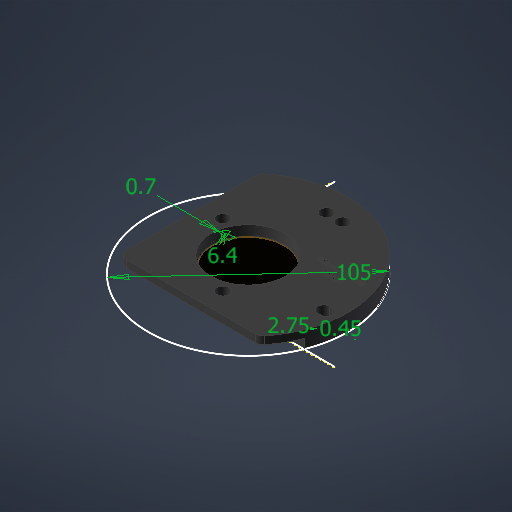
# Autodesk Inventor part: 40x4.35mm Coin Fixture Makera Air V2
Saved by Autodesk Inventor 2026.1 (Build 301233020, 233B)
## iProperties
Created: 2026-01-16
Part Number: 40x4.35mm Coin Fixture Makera Air V2
Material: Generic
Document SubType Name: Modeling
Designer: incep
Density: 1 g/cm^3
Appearance: Default
Author: incep
## iProperties of the stored document 40x4.35mm Coin Fixture Makera Air_3DPrint.ipt
Created: 2026-01-16
Part Number: 40x4.35mm Coin Fixture Makera Air_3DPrint
Material: Generic
Document SubType Name: Modeling
Designer: incep
Density: 1 g/cm^3
Appearance: Default
Author: incep
Autodesk Inventor part; units mm, degrees
ref_plane "YZ Plane" through (0, 0, 0) normal (1, 0, 0) x (0, 1, 0)
ref_plane "XZ Plane" through (0, 0, 0) normal (0, 1, 0) x (-1, 0, 0)
ref_plane "XY Plane" through (0, 0, 0) normal (0, 0, 1) x (1, 0, 0)
sketch "Sketch1" plane through (0, 0, 0) normal (0, 1, 0) x (-1, 0, 0)
  line L0 (0, -85) -> (15, -85) construction
  line L1 (15, -85) -> (15, 15) construction
  line L2 (15, 15) -> (-85, 15) construction
  line L3 (-85, 15) -> (-85, 0) construction
  arc A0 (0, -34.3692) -> (0, -25.6308) centre (3, -30) ccw construction
  arc A1 (-25.6308, 0) -> (-34.3692, 0) centre (-30, 3) ccw construction
  line L4 (0, 0) -> (0, -25.6308) construction
  line L5 (0, -34.3692) -> (0, -85) construction
  line L6 (-85, 0) -> (-34.3692, 0) construction
  line L7 (-25.6308, 0) -> (0, 0) construction
  circle A2 centre (-20.1, -20.1) radius 20.1 construction
  circle A3 centre (-30, -60) radius 1.375 construction
  circle A4 centre (-65, -15) radius 1.375 construction
  circle A5 centre (-66.5, -15) radius 1.375 construction
  circle A6 centre (-21.5, -60) radius 1.375 construction
  dimension "d0" = 85
  dimension "d1" = 15
  dimension "d2" = 100
  dimension "d3" = 100
  dimension "d4" = 15
  dimension "d5" = 85
  dimension "d6" = 10.6
  dimension "d7" = 3
  dimension "d8" = 30
  dimension "d9" = 10.6
  dimension "d10" = 3
  dimension "d11" = 30
  dimension "d12" = 40.2
  dimension "d13" = 2.75
  dimension "d14" = 2.75
  dimension "d15" = 30
  dimension "d16" = 60
  dimension "d17" = 65
  dimension "d18" = 15
  dimension "d49" = 2.75
  dimension "d50" = 2.75
  dimension "d51" = 18
  dimension "d52" = 36.5
  dimension "d53" = 8.5
  dimension "d54" = 63
  constraints: 16 end point, 7 centre point, 5 perpendicular, 4 point on circle, 2 collinear, 2 tangent, 2 vertical
  measures "d0" distance of L4.start L0.start
  measures "d1" distance of L0.start L0.end
  measures "d2" distance of L0.end L1.end
  measures "d3" distance of L1.end L2.end
  measures "d4" distance of L2.end L3.end
  measures "d5" distance of L3.end L4.start
  measures "d6" diameter of A0
  measures "d7" horizontal distance of L4.start A0.centre
  measures "d8" vertical distance of L4.start A0.centre
  measures "d9" diameter of A1
  measures "d10" vertical distance of A1.centre L4.start
  measures "d11" horizontal distance of A1.centre L4.start
  measures "d12" diameter of A2
  measures "d13" diameter of A3
  measures "d14" diameter of A4
  measures "d15" horizontal distance of L4.start A3.centre
  measures "d16" vertical distance of L4.start A3.centre
  measures "d17" horizontal distance of L4.start A4.centre
  measures "d18" vertical distance of L4.start A4.centre
  measures "d49" diameter of A5
  measures "d50" diameter of A6
  measures "d51" vertical distance of A5.centre A1.centre
  measures "d52" horizontal distance of A5.centre A1.centre
  measures "d53" horizontal distance of A1.centre A6.centre
  measures "d54" vertical distance of A1.centre A6.centre
sketch "Sketch2" plane through (0, 0, 0) normal (0, 1, 0) x (-1, 0, 0)
  line L0 (0, 0) -> (0, -25.6308) construction
  line L1 (-25.6308, 0) -> (0, 0) construction
  circle A0 centre (-20.1, -20.1) radius 20.1 projected
  arc A1 (-25.6308, 0) -> (-34.3692, 0) centre (-30, 3) ccw construction
  line L2 (-85, 0) -> (-34.3692, 0) construction
  arc A2 (0, -34.3692) -> (0, -25.6308) centre (3, -30) ccw construction
  line L3 (0, -34.3692) -> (0, -85) construction
  line L4 (-85, -0.7) -> (-32.7331, -0.7)
  arc A3 (-27.2669, -0.7) -> (-32.7331, -0.7) centre (-30, 3) ccw
  line L5 (-27.2669, -0.7) -> (-0.7, -0.7)
  line L6 (-0.7, -0.7) -> (-0.7, -27.2669)
  arc A4 (-0.7, -32.7331) -> (-0.7, -27.2669) centre (3, -30) ccw
  line L7 (-0.7, -32.7331) -> (-0.7, -85)
  circle A5 centre (-20.1, -20.1) radius 52.5
  circle A6 centre (-30, -60) radius 1.375 construction
  circle A7 centre (-65, -15) radius 1.375 construction
  circle A8 centre (3, -30) radius 3.2
  circle A9 centre (-30, 3) radius 3.2
  circle A10 centre (-65, -15) radius 3.2 construction
  circle A11 centre (-30, -60) radius 3.2
  circle A12 centre (-21.5, -60) radius 1.375 construction
  circle A13 centre (-66.5, -15) radius 1.375 construction
  circle A14 centre (-21.5, -60) radius 3.2
  line L8 (-65, -15) -> (-66.5, -15) construction
  line L9 (-65, -12.25) -> (-66.5, -12.25) construction
  line L10 (-66.5, -17.75) -> (-65, -17.75) construction
  arc A15 (-65, -17.75) -> (-65, -12.25) centre (-65, -15) ccw construction
  arc A16 (-66.5, -12.25) -> (-66.5, -17.75) centre (-66.5, -15) ccw construction
  line L11 (-66.5, -18.2) -> (-65, -18.2)
  arc A17 (-65, -18.2) -> (-65, -11.8) centre (-65, -15) ccw
  line L12 (-65, -11.8) -> (-66.5, -11.8)
  arc A18 (-66.5, -11.8) -> (-66.5, -18.2) centre (-66.5, -15) ccw
  point P0 (-0.7, -14.8417)
  point P1 (-14.8417, -0.7)
  point P2 (-68.8841, -0.7)
  point P3 (-0.7, -68.8841)
  point P4 (-0.7, -25.3583)
  point P5 (-25.3583, -0.7)
  point P6 (-65.75, -15)
  dimension "d19" = 0.7
  dimension "d20" = 6.4
  dimension "d24" = 105
  dimension "d55" = 2.75
  dimension "d56" = 0.45
  constraints: 20 end point, 12 centre point, 12 point on circle, 7 coincident, 4 equal radius, 4 tangent, 2 parallel, 1 horizontal, 1 midpoint, 8 other
  measures "d19" radial gap between concentric circles of A2 A4
  measures "d20" diameter of A8
  measures "d24" diameter of A5
  measures "d55" radius of A15
  measures "d56" radial gap between concentric circles of A16 A18
extrude "Extrusion1" add sketch "Sketch2" along normal blind 3.85 contours A0 L5 L6 | L6 A4 L7 A5 L4 A3 L5 A0 picked at (-4.2094, -4.2094) picked at (-56.8347, -28.8273)
sketch "Sketch3" plane through (0, 3.85, 0) normal (0, 1, 0) x (1, 0, 0)
  circle A0 centre (20.1, 20.1) radius 19
  arc A1 (25.3583, 0.7) -> (0.7, 25.3583) centre (20.1, 20.1) ccw projected
  circle A2 centre (30, 60) radius 1.375 construction
  circle A3 centre (65, 15) radius 1.375 construction
  circle A4 centre (-3, 30) radius 3.2 projected
  circle A5 centre (30, -3) radius 3.2 projected
  circle A6 centre (30, 60) radius 5.3
  circle A7 centre (65, 15) radius 5.3
  circle A8 centre (-3, 30) radius 5.3
  circle A9 centre (30, -3) radius 5.3
  arc A10 (0, 34.3692) -> (0, 25.6308) centre (-3, 30) ccw construction
  line L0 (32.7331, 0.7) -> (68.8841, 0.7) projected
  arc A11 (68.8841, 0.7) -> (0.7, 68.8841) centre (20.1, 20.1) ccw projected
  line L1 (0.7, 68.8841) -> (0.7, 32.7331) projected
  arc A12 (0.7, 32.7331) -> (0.7, 27.2669) centre (-3, 30) ccw projected
  line L2 (0.7, 27.2669) -> (0.7, 25.3583) projected
  arc A13 (25.3583, 0.7) -> (0.7, 25.3583) centre (20.1, 20.1) ccw projected
  line L3 (25.3583, 0.7) -> (27.2669, 0.7) projected
  arc A14 (27.2669, 0.7) -> (32.7331, 0.7) centre (30, -3) ccw projected
  circle A15 centre (30, 60) radius 3.2 projected
  circle A16 centre (30, -3) radius 3.2 projected
  circle A17 centre (-3, 30) radius 3.2 projected
  arc A18 (0.7, 14.8417) -> (14.8417, 0.7) centre (20.1, 20.1) ccw projected
  line L4 (0.7, 25.3583) -> (0.7, 14.8417)
  line L5 (25.3583, 0.7) -> (14.8417, 0.7)
  line L6 (0.7, 0.7) -> (14.8417, 0.7) projected
  arc A19 (0.7, 14.8417) -> (14.8417, 0.7) centre (20.1, 20.1) ccw projected
  line L7 (0.7, 14.8417) -> (0.7, 0.7) projected
  circle A20 centre (21.5, 60) radius 3.2 projected
  arc A21 (66.5, 11.8) -> (66.5, 18.2) centre (66.5, 15) ccw projected
  line L8 (65, 11.8) -> (66.5, 11.8) projected
  arc A22 (65, 18.2) -> (65, 11.8) centre (65, 15) ccw projected
  line L9 (65, 18.2) -> (66.5, 18.2) projected
  arc A23 (66.5, 11.8) -> (66.5, 18.2) centre (66.5, 15) ccw projected
  arc A24 (65, 18.2) -> (65, 11.8) centre (65, 15) ccw projected
  line L10 (32.7331, 0.7) -> (68.8841, 0.7) projected
  arc A25 (27.2669, 0.7) -> (32.7331, 0.7) centre (30, -3) ccw projected
  line L11 (25.3583, 0.7) -> (27.2669, 0.7) projected
  arc A26 (25.3583, 0.7) -> (0.7, 25.3583) centre (20.1, 20.1) ccw projected
  line L12 (0.7, 27.2669) -> (0.7, 25.3583) projected
  arc A27 (0.7, 32.7331) -> (0.7, 27.2669) centre (-3, 30) ccw projected
  line L13 (0.7, 68.8841) -> (0.7, 32.7331) projected
  arc A28 (68.8841, 0.7) -> (0.7, 68.8841) centre (20.1, 20.1) ccw projected
  arc A29 (66.5, 11.8) -> (66.5, 18.2) centre (66.5, 15) ccw projected
  line L14 (65, 18.2) -> (66.5, 18.2) projected
  arc A30 (65, 18.2) -> (65, 11.8) centre (65, 15) ccw projected
  line L15 (66.5, 11.8) -> (65, 11.8) projected
  circle A31 centre (21.5, 60) radius 3.2 projected
  circle A32 centre (30, 60) radius 3.2 projected
  circle A33 centre (30, -3) radius 3.2 projected
  circle A34 centre (-3, 30) radius 3.2 projected
  point P0 (0, 0)
  point P1 (0.7, 33.7947)
  point P2 (1.0901, 26.6293)
  point P3 (0.7, 25.3583)
  point P4 (25.3583, 0.7)
  point P5 (26.6293, 1.0901)
  point P6 (33.7947, 0.7)
  point P7 (69.3517, 11.9747)
  point P8 (69.9097, 16.9962)
  point P9 (0.7, 14.8417)
  point P10 (14.8417, 0.7)
  point P11 (26.2053, 0.7)
  point P12 (0.7, 26.2053)
  point P13 (0.7, 25.3583)
  point P14 (26.6293, 1.0901)
  point P15 (29.3628, 2.2616)
  point P16 (2.2616, 29.3628)
  point P17 (1.0901, 26.6293)
  point P18 (24.7, 60)
  dimension "d27" = 38
  constraints: 5 centre point, 5 coincident, 4 end point, 4 equal radius, 1 horizontal, 1 vertical
  measures "d27" diameter of A0
extrude "Extrusion2" add sketch "Sketch3" along normal blind 5 contours L5 A18 L4 A1 A8 A9 | A1 A9 L3 | A9 A1 | A1 A9 L0 A14 L3 | L6 L7 A18 | A1 A8 L1 A11 L0 A9 | A8 A1 | A1 A8 L2 A12 L1 | L2 A8 A1 | A6 | A7
chamfer "Chamfer1" [suppressed]
sketch "Sketch4" plane through (0, 8.85, 0) normal (0, 1, 0) x (1, 0, 0)
  line L0 (39.4462, 38.7056) -> (64.6246, 38.7056) construction
  line L1 (64.6246, 38.7056) -> (64.6246, 34.6573) construction
  line L2 (64.6246, 34.6573) -> (39.4462, 34.6573) construction
  line L3 (39.4462, 34.6573) -> (39.4462, 38.7056) construction
  line L4 (42.1949, 36.3448) -> (41.7893, 36.3448)
  line L5 (41.7893, 36.3448) -> (41.7893, 35.638)
  line L6 (41.7893, 35.638) -> (41.063, 35.638)
  line L7 (41.063, 35.638) -> (41.063, 36.3448)
  line L8 (41.063, 36.3448) -> (39.7418, 36.3448)
  line L9 (39.7418, 36.3448) -> (39.7418, 36.9034)
  line L10 (39.7418, 36.9034) -> (41.0388, 38.6425)
  line L11 (41.0388, 38.6425) -> (41.7893, 38.6425)
  line L12 (41.7893, 38.6425) -> (41.7893, 36.884)
  line L13 (41.7893, 36.884) -> (42.1949, 36.884)
  line L14 (42.1949, 36.884) -> (42.1949, 36.3448)
  line L15 (41.063, 36.884) -> (41.063, 37.9041)
  line L16 (41.063, 37.9041) -> (40.3028, 36.884)
  line L17 (40.3028, 36.884) -> (41.063, 36.884)
  spline S0 degree 2 poles (44.7452, 37.1439) (44.7452, 36.7553) (44.6213, 36.1723) (44.4829, 35.9756) knots 0 0 0 1 2 2 2
  spline S1 degree 2 poles (44.4829, 35.9756) (44.3469, 35.7813) (43.9072, 35.5821) (43.5915, 35.5821) knots 0 0 0 1 2 2 2
  spline S2 degree 2 poles (43.5915, 35.5821) (43.2733, 35.5821) (42.8361, 35.7813) (42.6977, 35.9805) knots 0 0 0 1 2 2 2
  spline S3 degree 2 poles (42.6977, 35.9805) (42.5592, 36.1772) (42.4353, 36.7553) (42.4353, 37.1439) knots 0 0 0 1 2 2 2
  spline S4 degree 2 poles (42.4353, 37.1439) (42.4353, 37.5422) (42.5592, 38.1057) (42.7001, 38.3097) knots 0 0 0 1 2 2 2
  spline S5 degree 2 poles (42.7001, 38.3097) (42.841, 38.5089) (43.2854, 38.7032) (43.5915, 38.7032) knots 0 0 0 1 2 2 2
  spline S6 degree 2 poles (43.5915, 38.7032) (43.9145, 38.7032) (44.3469, 38.4992) (44.4853, 38.2976) knots 0 0 0 1 2 2 2
  spline S7 degree 2 poles (44.4853, 38.2976) (44.6213, 38.1008) (44.7452, 37.5203) (44.7452, 37.1439) knots 0 0 0 1 2 2 2
  spline S8 degree 2 poles (43.9898, 37.1439) (43.9898, 37.7001) (43.8076, 38.1494) (43.5915, 38.1494) knots 0 0 0 1 2 2 2
  spline S9 degree 2 poles (43.5915, 38.1494) (43.3753, 38.1494) (43.1907, 37.7001) (43.1907, 37.1414) knots 0 0 0 1 2 2 2
  spline S10 degree 2 poles (43.1907, 37.1414) (43.1907, 36.5925) (43.3753, 36.1359) (43.5915, 36.1359) knots 0 0 0 1 2 2 2
  spline S11 degree 2 poles (43.5915, 36.1359) (43.8052, 36.1359) (43.9898, 36.5925) (43.9898, 37.1439) knots 0 0 0 1 2 2 2
  line L18 (47.4023, 35.6453) -> (46.5765, 35.6453)
  line L19 (46.5765, 35.6453) -> (46.1466, 36.2938)
  line L20 (46.1466, 36.2938) -> (45.7046, 35.6453)
  line L21 (45.7046, 35.6453) -> (44.8958, 35.6453)
  line L22 (44.8958, 35.6453) -> (45.7289, 36.7771)
  line L23 (45.7289, 36.7771) -> (44.9103, 37.9065)
  line L24 (44.9103, 37.9065) -> (45.7362, 37.9065)
  line L25 (45.7362, 37.9065) -> (46.1588, 37.2702)
  line L26 (46.1588, 37.2702) -> (46.5838, 37.9065)
  line L27 (46.5838, 37.9065) -> (47.3926, 37.9065)
  line L28 (47.3926, 37.9065) -> (46.5741, 36.7941)
  line L29 (46.5741, 36.7941) -> (47.4023, 35.6453)
  line L30 (49.9381, 36.3448) -> (49.5324, 36.3448)
  line L31 (49.5324, 36.3448) -> (49.5324, 35.638)
  line L32 (49.5324, 35.638) -> (48.8062, 35.638)
  line L33 (48.8062, 35.638) -> (48.8062, 36.3448)
  line L34 (48.8062, 36.3448) -> (47.4849, 36.3448)
  line L35 (47.4849, 36.3448) -> (47.4849, 36.9034)
  line L36 (47.4849, 36.9034) -> (48.7819, 38.6425)
  line L37 (48.7819, 38.6425) -> (49.5324, 38.6425)
  line L38 (49.5324, 38.6425) -> (49.5324, 36.884)
  line L39 (49.5324, 36.884) -> (49.9381, 36.884)
  line L40 (49.9381, 36.884) -> (49.9381, 36.3448)
  line L41 (48.8062, 36.884) -> (48.8062, 37.9041)
  line L42 (48.8062, 37.9041) -> (48.046, 36.884)
  line L43 (48.046, 36.884) -> (48.8062, 36.884)
  line L44 (51.0189, 35.6453) -> (50.3072, 35.6453)
  line L45 (50.3072, 35.6453) -> (50.3072, 36.4371)
  line L46 (50.3072, 36.4371) -> (51.0189, 36.4371)
  line L47 (51.0189, 36.4371) -> (51.0189, 35.6453)
  spline S12 degree 2 poles (53.7392, 36.5537) (53.7392, 36.3326) (53.5765, 35.9707) (53.4186, 35.8444) knots 0 0 0 1 2 2 2
  spline S13 degree 2 poles (53.4186, 35.8444) (53.2607, 35.7181) (52.8308, 35.5821) (52.5224, 35.5821) knots 0 0 0 1 2 2 2
  spline S14 degree 2 poles (52.5224, 35.5821) (52.1726, 35.5821) (51.6723, 35.6987) (51.5144, 35.7716) knots 0 0 0 1 2 2 2
  line L48 (51.5144, 35.7716) -> (51.5144, 36.4225)
  line L49 (51.5144, 36.4225) -> (51.5872, 36.4225)
  spline S15 degree 2 poles (51.5872, 36.4225) (51.7524, 36.3181) (52.1969, 36.1626) (52.3815, 36.1626) knots 0 0 0 1 2 2 2
  spline S16 degree 2 poles (52.3815, 36.1626) (52.4908, 36.1626) (52.7458, 36.2015) (52.8332, 36.2646) knots 0 0 0 1 2 2 2
  spline S17 degree 2 poles (52.8332, 36.2646) (52.9013, 36.3156) (52.9838, 36.4638) (52.9838, 36.5974) knots 0 0 0 1 2 2 2
  spline S18 degree 2 poles (52.9838, 36.5974) (52.9838, 36.731) (52.8673, 36.8743) (52.7701, 36.9083) knots 0 0 0 1 2 2 2
  spline S19 degree 2 poles (52.7701, 36.9083) (52.6729, 36.9423) (52.4033, 36.9496) (52.2989, 36.9496) knots 0 0 0 1 2 2 2
  line L50 (52.2989, 36.9496) -> (52.1702, 36.9496)
  line L51 (52.1702, 36.9496) -> (52.1702, 37.4766)
  line L52 (52.1702, 37.4766) -> (52.2892, 37.4766)
  spline S20 degree 2 poles (52.2892, 37.4766) (52.4252, 37.4766) (52.6559, 37.5009) (52.7361, 37.5374) knots 0 0 0 1 2 2 2
  spline S21 degree 2 poles (52.7361, 37.5374) (52.8162, 37.5762) (52.9061, 37.7122) (52.9061, 37.8288) knots 0 0 0 1 2 2 2
  spline S22 degree 2 poles (52.9061, 37.8288) (52.9061, 37.9211) (52.8211, 38.0353) (52.7604, 38.0668) knots 0 0 0 1 2 2 2
  spline S23 degree 2 poles (52.7604, 38.0668) (52.6875, 38.1033) (52.4932, 38.1276) (52.4252, 38.1276) knots 0 0 0 1 2 2 2
  spline S24 degree 2 poles (52.4252, 38.1276) (52.3159, 38.1276) (52.0852, 38.0766) (51.9783, 38.0353) knots 0 0 0 1 2 2 2
  spline S25 degree 2 poles (51.9783, 38.0353) (51.8933, 38.0037) (51.7087, 37.9017) (51.665, 37.875) knots 0 0 0 1 2 2 2
  line L53 (51.665, 37.875) -> (51.6018, 37.875)
  line L54 (51.6018, 37.875) -> (51.6018, 38.5162)
  spline S26 degree 2 poles (51.6018, 38.5162) (51.7573, 38.5818) (52.2819, 38.7056) (52.5564, 38.7056) knots 0 0 0 1 2 2 2
  spline S27 degree 2 poles (52.5564, 38.7056) (52.8235, 38.7056) (53.217, 38.6133) (53.3555, 38.5235) knots 0 0 0 1 2 2 2
  spline S28 degree 2 poles (53.3555, 38.5235) (53.5085, 38.4287) (53.6615, 38.1373) (53.6615, 37.9551) knots 0 0 0 1 2 2 2
  spline S29 degree 2 poles (53.6615, 37.9551) (53.6615, 37.6977) (53.3652, 37.3139) (53.1223, 37.258) knots 0 0 0 1 2 2 2
  line L55 (53.1223, 37.258) -> (53.1223, 37.2289)
  spline S30 degree 2 poles (53.1223, 37.2289) (53.2292, 37.2143) (53.4332, 37.1366) (53.5303, 37.0492) knots 0 0 0 1 2 2 2
  spline S31 degree 2 poles (53.5303, 37.0492) (53.6202, 36.9714) (53.7392, 36.7237) (53.7392, 36.5537) knots 0 0 0 1 2 2 2
  spline S32 degree 2 poles (56.3721, 36.6605) (56.3721, 36.4249) (56.2118, 36.0266) (56.0539, 35.8833) knots 0 0 0 1 2 2 2
  spline S33 degree 2 poles (56.0539, 35.8833) (55.896, 35.74) (55.4637, 35.5821) (55.1479, 35.5821) knots 0 0 0 1 2 2 2
  spline S34 degree 2 poles (55.1479, 35.5821) (54.8128, 35.5846) (54.3318, 35.6939) (54.174, 35.7643) knots 0 0 0 1 2 2 2
  line L56 (54.174, 35.7643) -> (54.174, 36.4177)
  line L57 (54.174, 36.4177) -> (54.242, 36.4177)
  spline S35 degree 2 poles (54.242, 36.4177) (54.3003, 36.3861) (54.4411, 36.3035) (54.5553, 36.2598) knots 0 0 0 1 2 2 2
  spline S36 degree 2 poles (54.5553, 36.2598) (54.6622, 36.2185) (54.8832, 36.1626) (55.0168, 36.1626) knots 0 0 0 1 2 2 2
  spline S37 degree 2 poles (55.0168, 36.1626) (55.1334, 36.1626) (55.4054, 36.2209) (55.488, 36.2986) knots 0 0 0 1 2 2 2
  spline S38 degree 2 poles (55.488, 36.2986) (55.5487, 36.3594) (55.6167, 36.5075) (55.6167, 36.6314) knots 0 0 0 1 2 2 2
  spline S39 degree 2 poles (55.6167, 36.6314) (55.6167, 36.7383) (55.5293, 36.8888) (55.4588, 36.935) knots 0 0 0 1 2 2 2
  spline S40 degree 2 poles (55.4588, 36.935) (55.3568, 37.003) (55.0654, 37.0419) (54.9609, 37.0419) knots 0 0 0 1 2 2 2
  spline S41 degree 2 poles (54.9609, 37.0419) (54.7958, 37.0419) (54.4824, 36.9884) (54.3683, 36.9593) knots 0 0 0 1 2 2 2
  line L58 (54.3683, 36.9593) -> (54.3027, 36.9593)
  line L59 (54.3027, 36.9593) -> (54.3027, 38.6425)
  line L60 (54.3027, 38.6425) -> (56.2895, 38.6425)
  line L61 (56.2895, 38.6425) -> (56.2895, 38.0766)
  line L62 (56.2895, 38.0766) -> (55.0144, 38.0766)
  line L63 (55.0144, 38.0766) -> (55.0144, 37.5786)
  spline S42 degree 2 poles (55.0144, 37.5786) (55.0751, 37.5835) (55.2427, 37.5884) (55.2888, 37.5884) knots 0 0 0 1 2 2 2
  spline S43 degree 2 poles (55.2888, 37.5884) (55.505, 37.5884) (55.8693, 37.5009) (56.0126, 37.4111) knots 0 0 0 1 2 2 2
  spline S44 degree 2 poles (56.0126, 37.4111) (56.1826, 37.2993) (56.3721, 36.9277) (56.3721, 36.6605) knots 0 0 0 1 2 2 2
  line L64 (59.5272, 35.6453) -> (59.5272, 36.7747)
  spline S45 degree 2 poles (59.5272, 36.7747) (59.5272, 36.9423) (59.515, 37.1706) (59.4859, 37.2435) knots 0 0 0 1 2 2 2
  spline S46 degree 2 poles (59.4859, 37.2435) (59.4543, 37.3163) (59.328, 37.3819) (59.2138, 37.3819) knots 0 0 0 1 2 2 2
  spline S47 degree 2 poles (59.2138, 37.3819) (59.1337, 37.3819) (58.9782, 37.3115) (58.8859, 37.2459) knots 0 0 0 1 2 2 2
  line L65 (58.8859, 37.2459) -> (58.8859, 35.6453)
  line L66 (58.8859, 35.6453) -> (58.1767, 35.6453)
  line L67 (58.1767, 35.6453) -> (58.1767, 36.7747)
  spline S48 degree 2 poles (58.1767, 36.7747) (58.1767, 36.9399) (58.1621, 37.1706) (58.133, 37.2435) knots 0 0 0 1 2 2 2
  spline S49 degree 2 poles (58.133, 37.2435) (58.1014, 37.3163) (57.9751, 37.3819) (57.861, 37.3819) knots 0 0 0 1 2 2 2
  spline S50 degree 2 poles (57.861, 37.3819) (57.776, 37.3819) (57.6084, 37.3018) (57.5306, 37.2459) knots 0 0 0 1 2 2 2
  line L68 (57.5306, 37.2459) -> (57.5306, 35.6453)
  line L69 (57.5306, 35.6453) -> (56.8263, 35.6453)
  line L70 (56.8263, 35.6453) -> (56.8263, 37.9065)
  line L71 (56.8263, 37.9065) -> (57.5306, 37.9065)
  line L72 (57.5306, 37.9065) -> (57.5306, 37.6564)
  spline S51 degree 2 poles (57.5306, 37.6564) (57.7031, 37.8021) (58.0116, 37.9673) (58.2034, 37.9673) knots 0 0 0 1 2 2 2
  spline S52 degree 2 poles (58.2034, 37.9673) (58.4099, 37.9673) (58.7256, 37.7705) (58.8082, 37.5738) knots 0 0 0 1 2 2 2
  spline S53 degree 2 poles (58.8082, 37.5738) (59.0098, 37.7632) (59.3693, 37.9673) (59.5539, 37.9673) knots 0 0 0 1 2 2 2
  spline S54 degree 2 poles (59.5539, 37.9673) (59.7118, 37.9673) (59.9619, 37.8677) (60.0469, 37.7657) knots 0 0 0 1 2 2 2
  spline S55 degree 2 poles (60.0469, 37.7657) (60.1417, 37.6564) (60.2364, 37.3576) (60.2364, 37.1172) knots 0 0 0 1 2 2 2
  line L73 (60.2364, 37.1172) -> (60.2364, 35.6453)
  line L74 (60.2364, 35.6453) -> (59.5272, 35.6453)
  line L75 (63.457, 35.6453) -> (63.457, 36.7747)
  spline S56 degree 2 poles (63.457, 36.7747) (63.457, 36.9423) (63.4449, 37.1706) (63.4157, 37.2435) knots 0 0 0 1 2 2 2
  spline S57 degree 2 poles (63.4157, 37.2435) (63.3842, 37.3163) (63.2579, 37.3819) (63.1437, 37.3819) knots 0 0 0 1 2 2 2
  spline S58 degree 2 poles (63.1437, 37.3819) (63.0636, 37.3819) (62.9081, 37.3115) (62.8158, 37.2459) knots 0 0 0 1 2 2 2
  line L76 (62.8158, 37.2459) -> (62.8158, 35.6453)
  line L77 (62.8158, 35.6453) -> (62.1066, 35.6453)
  line L78 (62.1066, 35.6453) -> (62.1066, 36.7747)
  spline S59 degree 2 poles (62.1066, 36.7747) (62.1066, 36.9399) (62.092, 37.1706) (62.0629, 37.2435) knots 0 0 0 1 2 2 2
  spline S60 degree 2 poles (62.0629, 37.2435) (62.0313, 37.3163) (61.905, 37.3819) (61.7908, 37.3819) knots 0 0 0 1 2 2 2
  spline S61 degree 2 poles (61.7908, 37.3819) (61.7058, 37.3819) (61.5382, 37.3018) (61.4605, 37.2459) knots 0 0 0 1 2 2 2
  line L79 (61.4605, 37.2459) -> (61.4605, 35.6453)
  line L80 (61.4605, 35.6453) -> (60.7562, 35.6453)
  line L81 (60.7562, 35.6453) -> (60.7562, 37.9065)
  line L82 (60.7562, 37.9065) -> (61.4605, 37.9065)
  line L83 (61.4605, 37.9065) -> (61.4605, 37.6564)
  spline S62 degree 2 poles (61.4605, 37.6564) (61.633, 37.8021) (61.9414, 37.9673) (62.1333, 37.9673) knots 0 0 0 1 2 2 2
  spline S63 degree 2 poles (62.1333, 37.9673) (62.3398, 37.9673) (62.6555, 37.7705) (62.7381, 37.5738) knots 0 0 0 1 2 2 2
  spline S64 degree 2 poles (62.7381, 37.5738) (62.9397, 37.7632) (63.2992, 37.9673) (63.4838, 37.9673) knots 0 0 0 1 2 2 2
  spline S65 degree 2 poles (63.4838, 37.9673) (63.6416, 37.9673) (63.8918, 37.8677) (63.9768, 37.7657) knots 0 0 0 1 2 2 2
  spline S66 degree 2 poles (63.9768, 37.7657) (64.0715, 37.6564) (64.1663, 37.3576) (64.1663, 37.1172) knots 0 0 0 1 2 2 2
  line L84 (64.1663, 37.1172) -> (64.1663, 35.6453)
  line L85 (64.1663, 35.6453) -> (63.457, 35.6453)
  spline S67 degree 2 poles (48.0909, 30.6522) (47.4157, 30.6522) (46.6239, 31.4683) (46.6239, 32.2066) knots 0 0 0 1 2 2 2
  spline S68 degree 2 poles (46.6239, 32.2066) (46.6239, 32.9183) (47.4181, 33.766) (48.0933, 33.766) knots 0 0 0 1 2 2 2
  spline S69 degree 2 poles (48.0933, 33.766) (48.2707, 33.766) (48.5573, 33.7247) (48.6884, 33.6907) knots 0 0 0 1 2 2 2
  spline S70 degree 2 poles (48.6884, 33.6907) (48.7904, 33.6591) (49.0309, 33.5546) (49.1062, 33.5158) knots 0 0 0 1 2 2 2
  line L86 (49.1062, 33.5158) -> (49.1062, 32.8017)
  line L87 (49.1062, 32.8017) -> (49.0309, 32.8017)
  spline S71 degree 2 poles (49.0309, 32.8017) (48.975, 32.8503) (48.8099, 32.9863) (48.7054, 33.0494) knots 0 0 0 1 2 2 2
  spline S72 degree 2 poles (48.7054, 33.0494) (48.601, 33.115) (48.3508, 33.2049) (48.2124, 33.2049) knots 0 0 0 1 2 2 2
  spline S73 degree 2 poles (48.2124, 33.2049) (48.0496, 33.2049) (47.78, 33.1029) (47.6562, 32.9742) knots 0 0 0 1 2 2 2
  spline S74 degree 2 poles (47.6562, 32.9742) (47.5444, 32.86) (47.4011, 32.469) (47.4011, 32.2042) knots 0 0 0 1 2 2 2
  spline S75 degree 2 poles (47.4011, 32.2042) (47.4011, 31.9249) (47.5493, 31.5436) (47.6707, 31.427) knots 0 0 0 1 2 2 2
  spline S76 degree 2 poles (47.6707, 31.427) (47.7873, 31.3128) (48.0739, 31.2132) (48.2172, 31.2132) knots 0 0 0 1 2 2 2
  spline S77 degree 2 poles (48.2172, 31.2132) (48.3654, 31.2132) (48.635, 31.3128) (48.7273, 31.3735) knots 0 0 0 1 2 2 2
  spline S78 degree 2 poles (48.7273, 31.3735) (48.8293, 31.4343) (48.9823, 31.563) (49.0382, 31.614) knots 0 0 0 1 2 2 2
  line L88 (49.0382, 31.614) -> (49.1062, 31.614)
  line L89 (49.1062, 31.614) -> (49.1062, 30.9096)
  spline S79 degree 2 poles (49.1062, 30.9096) (49.0236, 30.8708) (48.8074, 30.7736) (48.6908, 30.7396) knots 0 0 0 1 2 2 2
  spline S80 degree 2 poles (48.6908, 30.7396) (48.55, 30.6959) (48.3047, 30.6522) (48.0909, 30.6522) knots 0 0 0 1 2 2 2
  spline S81 degree 2 poles (52.2783, 32.2091) (52.2783, 31.4804) (51.501, 30.6473) (50.8258, 30.6473) knots 0 0 0 1 2 2 2
  spline S82 degree 2 poles (50.8258, 30.6473) (50.1482, 30.6473) (49.3758, 31.4901) (49.3758, 32.2091) knots 0 0 0 1 2 2 2
  spline S83 degree 2 poles (49.3758, 32.2091) (49.3758, 32.9304) (50.1482, 33.7708) (50.8258, 33.7708) knots 0 0 0 1 2 2 2
  spline S84 degree 2 poles (50.8258, 33.7708) (51.501, 33.7708) (52.2783, 32.9353) (52.2783, 32.2091) knots 0 0 0 1 2 2 2
  spline S85 degree 2 poles (51.501, 32.2091) (51.501, 32.4787) (51.3917, 32.8551) (51.297, 32.9742) knots 0 0 0 1 2 2 2
  spline S86 degree 2 poles (51.297, 32.9742) (51.2023, 33.098) (50.9594, 33.2049) (50.8282, 33.2049) knots 0 0 0 1 2 2 2
  spline S87 degree 2 poles (50.8282, 33.2049) (50.6898, 33.2049) (50.4639, 33.1053) (50.3595, 32.979) knots 0 0 0 1 2 2 2
  spline S88 degree 2 poles (50.3595, 32.979) (50.2672, 32.8624) (50.153, 32.4762) (50.153, 32.2091) knots 0 0 0 1 2 2 2
  spline S89 degree 2 poles (50.153, 32.2091) (50.153, 31.9322) (50.2623, 31.5679) (50.357, 31.444) knots 0 0 0 1 2 2 2
  spline S90 degree 2 poles (50.357, 31.444) (50.4518, 31.3201) (50.6971, 31.2132) (50.8282, 31.2132) knots 0 0 0 1 2 2 2
  spline S91 degree 2 poles (50.8282, 31.2132) (50.9618, 31.2132) (51.2096, 31.3274) (51.2994, 31.4488) knots 0 0 0 1 2 2 2
  spline S92 degree 2 poles (51.2994, 31.4488) (51.3966, 31.58) (51.501, 31.9273) (51.501, 32.2091) knots 0 0 0 1 2 2 2
  line L90 (54.2165, 30.7105) -> (52.6037, 30.7105)
  line L91 (52.6037, 30.7105) -> (52.6037, 31.2327)
  line L92 (52.6037, 31.2327) -> (53.0336, 31.2327)
  line L93 (53.0336, 31.2327) -> (53.0336, 33.1855)
  line L94 (53.0336, 33.1855) -> (52.6037, 33.1855)
  line L95 (52.6037, 33.1855) -> (52.6037, 33.7077)
  line L96 (52.6037, 33.7077) -> (54.2165, 33.7077)
  line L97 (54.2165, 33.7077) -> (54.2165, 33.1855)
  line L98 (54.2165, 33.1855) -> (53.7866, 33.1855)
  line L99 (53.7866, 33.1855) -> (53.7866, 31.2327)
  line L100 (53.7866, 31.2327) -> (54.2165, 31.2327)
  line L101 (54.2165, 31.2327) -> (54.2165, 30.7105)
  line L102 (57.2841, 30.7105) -> (56.5603, 30.7105)
  line L103 (56.5603, 30.7105) -> (55.4042, 32.7993)
  line L104 (55.4042, 32.7993) -> (55.4042, 30.7105)
  line L105 (55.4042, 30.7105) -> (54.7168, 30.7105)
  line L106 (54.7168, 30.7105) -> (54.7168, 33.7077)
  line L107 (54.7168, 33.7077) -> (55.6398, 33.7077)
  line L108 (55.6398, 33.7077) -> (56.5968, 31.9905)
  line L109 (56.5968, 31.9905) -> (56.5968, 33.7077)
  line L110 (56.5968, 33.7077) -> (57.2841, 33.7077)
  line L111 (57.2841, 33.7077) -> (57.2841, 30.7105)
  point P0 (0, 0)
  dimension "d0" = 85
  dimension "d1" = 15
  dimension "d2" = 100
  dimension "d3" = 100
  dimension "d4" = 15
  dimension "d5" = 85
  dimension "d6" = 10.6
  dimension "d7" = 3
  dimension "d8" = 30
  dimension "d9" = 10.6
  dimension "d10" = 3
  dimension "d11" = 30
  dimension "d12" = 40.2
  dimension "d49" = 2.75
  dimension "d50" = 2.75
  dimension "d51" = 18
  dimension "d52" = 36.5
  dimension "d53" = 8.5
  dimension "d54" = 63
  constraints: 2 other
extrude "Extrusion3" cut sketch "Sketch4" against normal blind 0.5
sketch "Sketch5" plane through (0, 8.85, 0) normal (0, 1, 0) x (1, 0, 0)
  line L0 (-15, 85) -> (-15, -15) projected
  line L1 (-15, -15) -> (85, -15) projected
  arc A0 (25.3583, 0.7) -> (0.7, 25.3583) centre (20.1, 20.1) ccw projected
  arc A1 (68.8841, 0.7) -> (0.7, 68.8841) centre (20.1, 20.1) ccw projected
  arc A2 (0.7, 68.8841) -> (-15, 59.1415) centre (20.1, 20.1) ccw
  circle A3 centre (-3, 30) radius 3.2 projected
  circle A4 centre (30, -3) radius 3.2 projected
  circle A5 centre (30, 60) radius 3.2 projected
  line L2 (32.7331, 0.7) -> (68.8841, 0.7) projected
  arc A6 (68.8841, 0.7) -> (0.7, 68.8841) centre (20.1, 20.1) ccw projected
  line L3 (0.7, 68.8841) -> (0.7, 32.7331) projected
  arc A7 (0.7, 32.7331) -> (0.7, 27.2669) centre (-3, 30) ccw projected
  line L4 (0.7, 27.2669) -> (0.7, 0.7) projected
  line L5 (0.7, 0.7) -> (27.2669, 0.7) projected
  arc A8 (27.2669, 0.7) -> (32.7331, 0.7) centre (30, -3) ccw projected
  arc A9 (59.1415, -15) -> (68.8841, 0.7) centre (20.1, 20.1) ccw
  line L6 (-14, 85) -> (-14, -14)
  line L7 (-14, -14) -> (85, -14)
  line L8 (0.7, 21.4274) -> (0.7, 18.7726)
  line L9 (14.8417, 0.7) -> (25.3583, 0.7) projected
  line L10 (21.4274, 0.7) -> (18.7726, 0.7)
  point P0 (0, 0)
  point P1 (0.7, 68.8841)
  point P2 (-14, 60.0179)
  point P3 (60.0179, -14)
  point P4 (21.4274, 0.7)
  point P5 (68.8841, 0.7)
  point P6 (0.7, 68.8841)
  dimension "d45" = 1
  constraints: 8 end point, 4 point on circle, 3 point on line, 2 centre point, 1 coincident, 1 collinear, 1 vertical, 1 other
  measures "d45" distance between parallel lines of L0 L6
extrude "Extrusion4" add sketch "Sketch5" against normal blind 4 contours A2 L3 A7 L4 L5 A8 L2 A9 L7 L6
fillet "Fillet1" radius 4 3 edges at (-14, 6.85, 14) (-14, 6.85, -60.0179) (60.0179, 6.85, 14)
ref_plane "Work Plane1" through (0, -0.45, 0) normal (0, -1, 0) x (1, 0, 0)
sketch "Sketch6" plane through (0, -0.45, 0) normal (0, -1, 0) x (1, 0, 0)
  circle A0 centre (20.1, -20.1) radius 20
  point P0 (0, 0)
  dimension "d39" = 40
  constraints: 1 centre point, 1 coincident
  measures "d39" diameter of A0
extrude "Extrusion5" add sketch "Sketch6" against normal blind 4.3 separate body
sketch "Sketch7" plane through (20.1, 3.85, -20.1) normal (0, 1, 0) x (1, 0, 0)
  circle A0 centre (0, 0) radius 20 projected
  circle A1 centre (0, 0) radius 18.75
  point P0 (-20.1, -20.1)
  dimension "d42" = 37.5
  constraints: 1 centre point, 1 coincident
  measures "d42" diameter of A1
extrude "Extrusion6" cut sketch "Sketch7" against normal blind 0.25 contours A1 bodies 2
chamfer "Chamfer2" distance 5 angle 5.09 1 edges at (1.1, 8.85, -20.1) measured on face at (39.0384, 7.1833, -18.5711)
body "Solid1"
